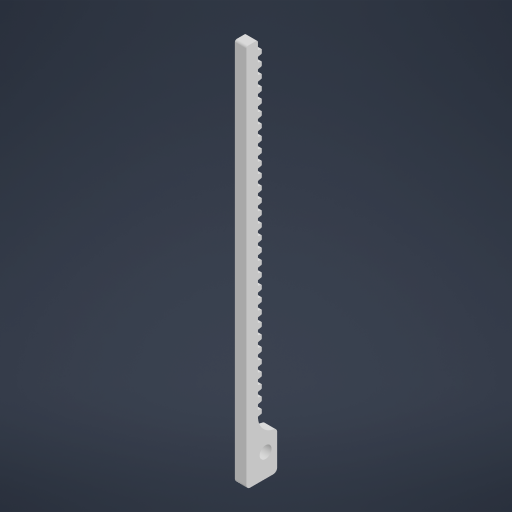
# Autodesk Inventor part: CamPole
Saved by Autodesk Inventor 2023 (Build 270158000, 158)
## iProperties
Created: 2023-03-14
Part Number: CamPole
Material: Generic
Document SubType Name: Modeling
Designer: Matt
Density: 1 g/cm^3
Appearance: Default
Author: Matt
Autodesk Inventor part; units mm, degrees
ref_plane "YZ Plane" through (0, 0, 0) normal (1, 0, 0) x (0, 1, 0)
ref_plane "XZ Plane" through (0, 0, 0) normal (0, 1, 0) x (-1, 0, 0)
ref_plane "XY Plane" through (0, 0, 0) normal (0, 0, 1) x (1, 0, 0)
sketch "Sketch1" plane through (0, 0, 0) normal (1, 0, 0) x (0, 1, 0)
  line L0 (0, 0) -> (10, 0)
  line L1 (10, 0) -> (10, -8)
  line L2 (10, -8) -> (0, -8)
  line L3 (0, -8) -> (0, 0)
  line L4 (10, 0) -> (100, 0)
  line L5 (100, 0) -> (100, -3)
  line L6 (100, -3) -> (10, -3)
  line L7 (10, -3) -> (10, 0)
  circle A0 centre (6, -5) radius 1.55
  dimension "d0" = 10
  dimension "d1" = 8
  dimension "d2" = 90
  dimension "d3" = 3
  dimension "d6" = 3.1
  dimension "d7" = 5
  dimension "d8" = 4
  constraints: 16 end point, 4 parallel, 2 horizontal, 2 perpendicular, 1 centre point
  measures "d0" distance of L1.end L2.end
  measures "d1" distance of L0.end L1.end
  measures "d2" distance of L0.end L4.end
  measures "d3" distance of L4.end L5.end
  measures "d6" diameter of A0
  measures "d7" distance from line of L0 A0.centre
  measures "d8" distance from line of L1 A0.centre
extrude "Extrusion1" add sketch "Sketch1" along normal blind 3
fillet "Fillet1" radius 5 1 edges at (1.5, 10, -3)
fillet "Fillet1" radius 1 3 edges at (1.5, 10, -8) (1.5, 0, 0) (1.5, 0, -8)
fillet "Fillet1" radius 0.5 2 edges at (1.5, 100, -3) (1.5, 100, 0)
sketch "Sketch3" plane through (3, 0, 0) normal (1, 0, 0) x (0, 0, -1)
  arc A0 (3, 15) -> (7.1667, 10.0699) centre (8, 15) ccw projected
  line L0 (3, 15) -> (4, 15)
  line L1 (4, 15) -> (4, 15.75)
  line L2 (4, 15.75) -> (3, 15.75)
  line L3 (3, 15) -> (3, 99.5) projected
  line L4 (3, 15) -> (3, 15.75)
  line L5 (4, 15) -> (4, 15.2)
  line L6 (4, 15.2) -> (3, 15)
  line L7 (3, 15) -> (3.1, 15)
  line L8 (3.1, 15) -> (3.1, 14.9)
  line L9 (3.1, 14.9) -> (3, 14.9)
  line L10 (3, 14.9) -> (3, 15)
  arc A1 (3.0995, 15.0199) -> (3, 14.9) centre (3.1238, 14.8985) ccw
  arc A2 (3.899, 15.1798) -> (4, 15.3306) centre (3.837, 15.3306) ccw
  line L11 (4, 15.3306) -> (4, 15.75)
  line L12 (3, 14.9) -> (3, 15.75)
  line L13 (3.899, 15.1798) -> (3.0995, 15.0199)
  line L14 (3, 16.5) -> (3, 15.75)
  line L15 (3, 16.6) -> (3, 16.5)
  arc A3 (3, 16.6) -> (3.0995, 16.4801) centre (3.1238, 16.6015) ccw
  arc A4 (4, 16.1694) -> (3.899, 16.3202) centre (3.837, 16.1694) ccw
  line L16 (4, 16.1694) -> (4, 15.75)
  line L17 (3.899, 16.3202) -> (3.0995, 16.4801)
  line L18 (4, 18.9694) -> (4, 18.55)
  arc A5 (3.899, 17.9798) -> (4, 18.1306) centre (3.837, 18.1306) ccw
  line L19 (3.899, 19.1202) -> (3.0995, 19.2801)
  arc A6 (4, 18.9694) -> (3.899, 19.1202) centre (3.837, 18.9694) ccw
  arc A7 (3, 19.4) -> (3.0995, 19.2801) centre (3.1238, 19.4015) ccw
  line L20 (3, 19.3) -> (3, 18.55)
  line L21 (3, 19.4) -> (3, 19.3)
  line L22 (3, 17.8) -> (3, 18.55)
  line L23 (3, 17.7) -> (3, 18.55)
  arc A8 (3.0995, 17.8199) -> (3, 17.7) centre (3.1238, 17.6985) ccw
  line L24 (4, 18.1306) -> (4, 18.55)
  line L25 (3.899, 17.9798) -> (3.0995, 17.8199)
  line L26 (4, 21.7694) -> (4, 21.35)
  arc A9 (3.899, 20.7798) -> (4, 20.9306) centre (3.837, 20.9306) ccw
  line L27 (3.899, 21.9202) -> (3.0995, 22.0801)
  arc A10 (4, 21.7694) -> (3.899, 21.9202) centre (3.837, 21.7694) ccw
  arc A11 (3, 22.2) -> (3.0995, 22.0801) centre (3.1238, 22.2015) ccw
  line L28 (3, 22.1) -> (3, 21.35)
  line L29 (3, 22.2) -> (3, 22.1)
  line L30 (3, 20.6) -> (3, 21.35)
  line L31 (3, 20.5) -> (3, 21.35)
  arc A12 (3.0995, 20.6199) -> (3, 20.5) centre (3.1238, 20.4985) ccw
  line L32 (4, 20.9306) -> (4, 21.35)
  line L33 (3.899, 20.7798) -> (3.0995, 20.6199)
  line L34 (4, 24.5694) -> (4, 24.15)
  arc A13 (3.899, 23.5798) -> (4, 23.7306) centre (3.837, 23.7306) ccw
  line L35 (3.899, 24.7202) -> (3.0995, 24.8801)
  arc A14 (4, 24.5694) -> (3.899, 24.7202) centre (3.837, 24.5694) ccw
  arc A15 (3, 25) -> (3.0995, 24.8801) centre (3.1238, 25.0015) ccw
  line L36 (3, 24.9) -> (3, 24.15)
  line L37 (3, 25) -> (3, 24.9)
  line L38 (3, 23.4) -> (3, 24.15)
  line L39 (3, 23.3) -> (3, 24.15)
  arc A16 (3.0995, 23.4199) -> (3, 23.3) centre (3.1238, 23.2985) ccw
  line L40 (4, 23.7306) -> (4, 24.15)
  line L41 (3.899, 23.5798) -> (3.0995, 23.4199)
  line L42 (4, 27.3694) -> (4, 26.95)
  arc A17 (3.899, 26.3798) -> (4, 26.5306) centre (3.837, 26.5306) ccw
  line L43 (3.899, 27.5202) -> (3.0995, 27.6801)
  arc A18 (4, 27.3694) -> (3.899, 27.5202) centre (3.837, 27.3694) ccw
  arc A19 (3, 27.8) -> (3.0995, 27.6801) centre (3.1238, 27.8015) ccw
  line L44 (3, 27.7) -> (3, 26.95)
  line L45 (3, 27.8) -> (3, 27.7)
  line L46 (3, 26.2) -> (3, 26.95)
  line L47 (3, 26.1) -> (3, 26.95)
  arc A20 (3.0995, 26.2199) -> (3, 26.1) centre (3.1238, 26.0985) ccw
  line L48 (4, 26.5306) -> (4, 26.95)
  line L49 (3.899, 26.3798) -> (3.0995, 26.2199)
  line L50 (4, 30.1694) -> (4, 29.75)
  arc A21 (3.899, 29.1798) -> (4, 29.3306) centre (3.837, 29.3306) ccw
  line L51 (3.899, 30.3202) -> (3.0995, 30.4801)
  arc A22 (4, 30.1694) -> (3.899, 30.3202) centre (3.837, 30.1694) ccw
  arc A23 (3, 30.6) -> (3.0995, 30.4801) centre (3.1238, 30.6015) ccw
  line L52 (3, 30.5) -> (3, 29.75)
  line L53 (3, 30.6) -> (3, 30.5)
  line L54 (3, 29) -> (3, 29.75)
  line L55 (3, 28.9) -> (3, 29.75)
  arc A24 (3.0995, 29.0199) -> (3, 28.9) centre (3.1238, 28.8985) ccw
  line L56 (4, 29.3306) -> (4, 29.75)
  line L57 (3.899, 29.1798) -> (3.0995, 29.0199)
  line L58 (4, 32.9694) -> (4, 32.55)
  arc A25 (3.899, 31.9798) -> (4, 32.1306) centre (3.837, 32.1306) ccw
  line L59 (3.899, 33.1202) -> (3.0995, 33.2801)
  arc A26 (4, 32.9694) -> (3.899, 33.1202) centre (3.837, 32.9694) ccw
  arc A27 (3, 33.4) -> (3.0995, 33.2801) centre (3.1238, 33.4015) ccw
  line L60 (3, 33.3) -> (3, 32.55)
  line L61 (3, 33.4) -> (3, 33.3)
  line L62 (3, 31.8) -> (3, 32.55)
  line L63 (3, 31.7) -> (3, 32.55)
  arc A28 (3.0995, 31.8199) -> (3, 31.7) centre (3.1238, 31.6985) ccw
  line L64 (4, 32.1306) -> (4, 32.55)
  line L65 (3.899, 31.9798) -> (3.0995, 31.8199)
  line L66 (4, 35.7694) -> (4, 35.35)
  arc A29 (3.899, 34.7798) -> (4, 34.9306) centre (3.837, 34.9306) ccw
  line L67 (3.899, 35.9202) -> (3.0995, 36.0801)
  arc A30 (4, 35.7694) -> (3.899, 35.9202) centre (3.837, 35.7694) ccw
  arc A31 (3, 36.2) -> (3.0995, 36.0801) centre (3.1238, 36.2015) ccw
  line L68 (3, 36.1) -> (3, 35.35)
  line L69 (3, 36.2) -> (3, 36.1)
  line L70 (3, 34.6) -> (3, 35.35)
  line L71 (3, 34.5) -> (3, 35.35)
  arc A32 (3.0995, 34.6199) -> (3, 34.5) centre (3.1238, 34.4985) ccw
  line L72 (4, 34.9306) -> (4, 35.35)
  line L73 (3.899, 34.7798) -> (3.0995, 34.6199)
  line L74 (4, 38.5694) -> (4, 38.15)
  arc A33 (3.899, 37.5798) -> (4, 37.7306) centre (3.837, 37.7306) ccw
  line L75 (3.899, 38.7202) -> (3.0995, 38.8801)
  arc A34 (4, 38.5694) -> (3.899, 38.7202) centre (3.837, 38.5694) ccw
  arc A35 (3, 39) -> (3.0995, 38.8801) centre (3.1238, 39.0015) ccw
  line L76 (3, 38.9) -> (3, 38.15)
  line L77 (3, 39) -> (3, 38.9)
  line L78 (3, 37.4) -> (3, 38.15)
  line L79 (3, 37.3) -> (3, 38.15)
  arc A36 (3.0995, 37.4199) -> (3, 37.3) centre (3.1238, 37.2985) ccw
  line L80 (4, 37.7306) -> (4, 38.15)
  line L81 (3.899, 37.5798) -> (3.0995, 37.4199)
  line L82 (4, 41.3694) -> (4, 40.95)
  arc A37 (3.899, 40.3798) -> (4, 40.5306) centre (3.837, 40.5306) ccw
  line L83 (3.899, 41.5202) -> (3.0995, 41.6801)
  arc A38 (4, 41.3694) -> (3.899, 41.5202) centre (3.837, 41.3694) ccw
  arc A39 (3, 41.8) -> (3.0995, 41.6801) centre (3.1238, 41.8015) ccw
  line L84 (3, 41.7) -> (3, 40.95)
  line L85 (3, 41.8) -> (3, 41.7)
  line L86 (3, 40.2) -> (3, 40.95)
  line L87 (3, 40.1) -> (3, 40.95)
  arc A40 (3.0995, 40.2199) -> (3, 40.1) centre (3.1238, 40.0985) ccw
  line L88 (4, 40.5306) -> (4, 40.95)
  line L89 (3.899, 40.3798) -> (3.0995, 40.2199)
  line L90 (4, 44.1694) -> (4, 43.75)
  arc A41 (3.899, 43.1798) -> (4, 43.3306) centre (3.837, 43.3306) ccw
  line L91 (3.899, 44.3202) -> (3.0995, 44.4801)
  arc A42 (4, 44.1694) -> (3.899, 44.3202) centre (3.837, 44.1694) ccw
  arc A43 (3, 44.6) -> (3.0995, 44.4801) centre (3.1238, 44.6015) ccw
  line L92 (3, 44.5) -> (3, 43.75)
  line L93 (3, 44.6) -> (3, 44.5)
  line L94 (3, 43) -> (3, 43.75)
  line L95 (3, 42.9) -> (3, 43.75)
  arc A44 (3.0995, 43.0199) -> (3, 42.9) centre (3.1238, 42.8985) ccw
  line L96 (4, 43.3306) -> (4, 43.75)
  line L97 (3.899, 43.1798) -> (3.0995, 43.0199)
  line L98 (4, 46.9694) -> (4, 46.55)
  arc A45 (3.899, 45.9798) -> (4, 46.1306) centre (3.837, 46.1306) ccw
  line L99 (3.899, 47.1202) -> (3.0995, 47.2801)
  arc A46 (4, 46.9694) -> (3.899, 47.1202) centre (3.837, 46.9694) ccw
  arc A47 (3, 47.4) -> (3.0995, 47.2801) centre (3.1238, 47.4015) ccw
  line L100 (3, 47.3) -> (3, 46.55)
  line L101 (3, 47.4) -> (3, 47.3)
  line L102 (3, 45.8) -> (3, 46.55)
  line L103 (3, 45.7) -> (3, 46.55)
  arc A48 (3.0995, 45.8199) -> (3, 45.7) centre (3.1238, 45.6985) ccw
  line L104 (4, 46.1306) -> (4, 46.55)
  line L105 (3.899, 45.9798) -> (3.0995, 45.8199)
  line L106 (4, 49.7694) -> (4, 49.35)
  arc A49 (3.899, 48.7798) -> (4, 48.9306) centre (3.837, 48.9306) ccw
  line L107 (3.899, 49.9202) -> (3.0995, 50.0801)
  arc A50 (4, 49.7694) -> (3.899, 49.9202) centre (3.837, 49.7694) ccw
  arc A51 (3, 50.2) -> (3.0995, 50.0801) centre (3.1238, 50.2015) ccw
  line L108 (3, 50.1) -> (3, 49.35)
  line L109 (3, 50.2) -> (3, 50.1)
  line L110 (3, 48.6) -> (3, 49.35)
  line L111 (3, 48.5) -> (3, 49.35)
  arc A52 (3.0995, 48.6199) -> (3, 48.5) centre (3.1238, 48.4985) ccw
  line L112 (4, 48.9306) -> (4, 49.35)
  line L113 (3.899, 48.7798) -> (3.0995, 48.6199)
  line L114 (4, 52.5694) -> (4, 52.15)
  arc A53 (3.899, 51.5798) -> (4, 51.7306) centre (3.837, 51.7306) ccw
  line L115 (3.899, 52.7202) -> (3.0995, 52.8801)
  arc A54 (4, 52.5694) -> (3.899, 52.7202) centre (3.837, 52.5694) ccw
  arc A55 (3, 53) -> (3.0995, 52.8801) centre (3.1238, 53.0015) ccw
  line L116 (3, 52.9) -> (3, 52.15)
  line L117 (3, 53) -> (3, 52.9)
  line L118 (3, 51.4) -> (3, 52.15)
  line L119 (3, 51.3) -> (3, 52.15)
  arc A56 (3.0995, 51.4199) -> (3, 51.3) centre (3.1238, 51.2985) ccw
  line L120 (4, 51.7306) -> (4, 52.15)
  line L121 (3.899, 51.5798) -> (3.0995, 51.4199)
  line L122 (4, 55.3694) -> (4, 54.95)
  arc A57 (3.899, 54.3798) -> (4, 54.5306) centre (3.837, 54.5306) ccw
  line L123 (3.899, 55.5202) -> (3.0995, 55.6801)
  arc A58 (4, 55.3694) -> (3.899, 55.5202) centre (3.837, 55.3694) ccw
  arc A59 (3, 55.8) -> (3.0995, 55.6801) centre (3.1238, 55.8015) ccw
  line L124 (3, 55.7) -> (3, 54.95)
  line L125 (3, 55.8) -> (3, 55.7)
  line L126 (3, 54.2) -> (3, 54.95)
  line L127 (3, 54.1) -> (3, 54.95)
  arc A60 (3.0995, 54.2199) -> (3, 54.1) centre (3.1238, 54.0985) ccw
  line L128 (4, 54.5306) -> (4, 54.95)
  line L129 (3.899, 54.3798) -> (3.0995, 54.2199)
  line L130 (4, 58.1694) -> (4, 57.75)
  arc A61 (3.899, 57.1798) -> (4, 57.3306) centre (3.837, 57.3306) ccw
  line L131 (3.899, 58.3202) -> (3.0995, 58.4801)
  arc A62 (4, 58.1694) -> (3.899, 58.3202) centre (3.837, 58.1694) ccw
  arc A63 (3, 58.6) -> (3.0995, 58.4801) centre (3.1238, 58.6015) ccw
  line L132 (3, 58.5) -> (3, 57.75)
  line L133 (3, 58.6) -> (3, 58.5)
  line L134 (3, 57) -> (3, 57.75)
  line L135 (3, 56.9) -> (3, 57.75)
  arc A64 (3.0995, 57.0199) -> (3, 56.9) centre (3.1238, 56.8985) ccw
  line L136 (4, 57.3306) -> (4, 57.75)
  line L137 (3.899, 57.1798) -> (3.0995, 57.0199)
  line L138 (4, 60.9694) -> (4, 60.55)
  arc A65 (3.899, 59.9798) -> (4, 60.1306) centre (3.837, 60.1306) ccw
  line L139 (3.899, 61.1202) -> (3.0995, 61.2801)
  arc A66 (4, 60.9694) -> (3.899, 61.1202) centre (3.837, 60.9694) ccw
  arc A67 (3, 61.4) -> (3.0995, 61.2801) centre (3.1238, 61.4015) ccw
  line L140 (3, 61.3) -> (3, 60.55)
  line L141 (3, 61.4) -> (3, 61.3)
  line L142 (3, 59.8) -> (3, 60.55)
  line L143 (3, 59.7) -> (3, 60.55)
  arc A68 (3.0995, 59.8199) -> (3, 59.7) centre (3.1238, 59.6985) ccw
  line L144 (4, 60.1306) -> (4, 60.55)
  line L145 (3.899, 59.9798) -> (3.0995, 59.8199)
  line L146 (4, 63.7694) -> (4, 63.35)
  arc A69 (3.899, 62.7798) -> (4, 62.9306) centre (3.837, 62.9306) ccw
  line L147 (3.899, 63.9202) -> (3.0995, 64.0801)
  arc A70 (4, 63.7694) -> (3.899, 63.9202) centre (3.837, 63.7694) ccw
  arc A71 (3, 64.2) -> (3.0995, 64.0801) centre (3.1238, 64.2015) ccw
  line L148 (3, 64.1) -> (3, 63.35)
  line L149 (3, 64.2) -> (3, 64.1)
  line L150 (3, 62.6) -> (3, 63.35)
  line L151 (3, 62.5) -> (3, 63.35)
  arc A72 (3.0995, 62.6199) -> (3, 62.5) centre (3.1238, 62.4985) ccw
  line L152 (4, 62.9306) -> (4, 63.35)
  line L153 (3.899, 62.7798) -> (3.0995, 62.6199)
  line L154 (4, 66.5694) -> (4, 66.15)
  arc A73 (3.899, 65.5798) -> (4, 65.7306) centre (3.837, 65.7306) ccw
  line L155 (3.899, 66.7202) -> (3.0995, 66.8801)
  arc A74 (4, 66.5694) -> (3.899, 66.7202) centre (3.837, 66.5694) ccw
  arc A75 (3, 67) -> (3.0995, 66.8801) centre (3.1238, 67.0015) ccw
  line L156 (3, 66.9) -> (3, 66.15)
  line L157 (3, 67) -> (3, 66.9)
  line L158 (3, 65.4) -> (3, 66.15)
  line L159 (3, 65.3) -> (3, 66.15)
  arc A76 (3.0995, 65.4199) -> (3, 65.3) centre (3.1238, 65.2985) ccw
  line L160 (4, 65.7306) -> (4, 66.15)
  line L161 (3.899, 65.5798) -> (3.0995, 65.4199)
  line L162 (4, 69.3694) -> (4, 68.95)
  arc A77 (3.899, 68.3798) -> (4, 68.5306) centre (3.837, 68.5306) ccw
  line L163 (3.899, 69.5202) -> (3.0995, 69.6801)
  arc A78 (4, 69.3694) -> (3.899, 69.5202) centre (3.837, 69.3694) ccw
  arc A79 (3, 69.8) -> (3.0995, 69.6801) centre (3.1238, 69.8015) ccw
  line L164 (3, 69.7) -> (3, 68.95)
  line L165 (3, 69.8) -> (3, 69.7)
  line L166 (3, 68.2) -> (3, 68.95)
  line L167 (3, 68.1) -> (3, 68.95)
  arc A80 (3.0995, 68.2199) -> (3, 68.1) centre (3.1238, 68.0985) ccw
  line L168 (4, 68.5306) -> (4, 68.95)
  line L169 (3.899, 68.3798) -> (3.0995, 68.2199)
  line L170 (4, 72.1694) -> (4, 71.75)
  arc A81 (3.899, 71.1798) -> (4, 71.3306) centre (3.837, 71.3306) ccw
  line L171 (3.899, 72.3202) -> (3.0995, 72.4801)
  arc A82 (4, 72.1694) -> (3.899, 72.3202) centre (3.837, 72.1694) ccw
  arc A83 (3, 72.6) -> (3.0995, 72.4801) centre (3.1238, 72.6015) ccw
  line L172 (3, 72.5) -> (3, 71.75)
  line L173 (3, 72.6) -> (3, 72.5)
  line L174 (3, 71) -> (3, 71.75)
  line L175 (3, 70.9) -> (3, 71.75)
  arc A84 (3.0995, 71.0199) -> (3, 70.9) centre (3.1238, 70.8985) ccw
  line L176 (4, 71.3306) -> (4, 71.75)
  line L177 (3.899, 71.1798) -> (3.0995, 71.0199)
  line L178 (4, 74.9694) -> (4, 74.55)
  arc A85 (3.899, 73.9798) -> (4, 74.1306) centre (3.837, 74.1306) ccw
  line L179 (3.899, 75.1202) -> (3.0995, 75.2801)
  arc A86 (4, 74.9694) -> (3.899, 75.1202) centre (3.837, 74.9694) ccw
  arc A87 (3, 75.4) -> (3.0995, 75.2801) centre (3.1238, 75.4015) ccw
  line L180 (3, 75.3) -> (3, 74.55)
  line L181 (3, 75.4) -> (3, 75.3)
  line L182 (3, 73.8) -> (3, 74.55)
  line L183 (3, 73.7) -> (3, 74.55)
  arc A88 (3.0995, 73.8199) -> (3, 73.7) centre (3.1238, 73.6985) ccw
  line L184 (4, 74.1306) -> (4, 74.55)
  line L185 (3.899, 73.9798) -> (3.0995, 73.8199)
  line L186 (4, 77.7694) -> (4, 77.35)
  arc A89 (3.899, 76.7798) -> (4, 76.9306) centre (3.837, 76.9306) ccw
  line L187 (3.899, 77.9202) -> (3.0995, 78.0801)
  arc A90 (4, 77.7694) -> (3.899, 77.9202) centre (3.837, 77.7694) ccw
  arc A91 (3, 78.2) -> (3.0995, 78.0801) centre (3.1238, 78.2015) ccw
  line L188 (3, 78.1) -> (3, 77.35)
  line L189 (3, 78.2) -> (3, 78.1)
  line L190 (3, 76.6) -> (3, 77.35)
  line L191 (3, 76.5) -> (3, 77.35)
  arc A92 (3.0995, 76.6199) -> (3, 76.5) centre (3.1238, 76.4985) ccw
  line L192 (4, 76.9306) -> (4, 77.35)
  line L193 (3.899, 76.7798) -> (3.0995, 76.6199)
  line L194 (4, 80.5694) -> (4, 80.15)
  arc A93 (3.899, 79.5798) -> (4, 79.7306) centre (3.837, 79.7306) ccw
  line L195 (3.899, 80.7202) -> (3.0995, 80.8801)
  arc A94 (4, 80.5694) -> (3.899, 80.7202) centre (3.837, 80.5694) ccw
  arc A95 (3, 81) -> (3.0995, 80.8801) centre (3.1238, 81.0015) ccw
  line L196 (3, 80.9) -> (3, 80.15)
  line L197 (3, 81) -> (3, 80.9)
  line L198 (3, 79.4) -> (3, 80.15)
  line L199 (3, 79.3) -> (3, 80.15)
  arc A96 (3.0995, 79.4199) -> (3, 79.3) centre (3.1238, 79.2985) ccw
  line L200 (4, 79.7306) -> (4, 80.15)
  line L201 (3.899, 79.5798) -> (3.0995, 79.4199)
  line L202 (4, 83.3694) -> (4, 82.95)
  arc A97 (3.899, 82.3798) -> (4, 82.5306) centre (3.837, 82.5306) ccw
  line L203 (3.899, 83.5202) -> (3.0995, 83.6801)
  arc A98 (4, 83.3694) -> (3.899, 83.5202) centre (3.837, 83.3694) ccw
  arc A99 (3, 83.8) -> (3.0995, 83.6801) centre (3.1238, 83.8015) ccw
  line L204 (3, 83.7) -> (3, 82.95)
  line L205 (3, 83.8) -> (3, 83.7)
  line L206 (3, 82.2) -> (3, 82.95)
  line L207 (3, 82.1) -> (3, 82.95)
  arc A100 (3.0995, 82.2199) -> (3, 82.1) centre (3.1238, 82.0985) ccw
  line L208 (4, 82.5306) -> (4, 82.95)
  line L209 (3.899, 82.3798) -> (3.0995, 82.2199)
  line L210 (4, 86.1694) -> (4, 85.75)
  arc A101 (3.899, 85.1798) -> (4, 85.3306) centre (3.837, 85.3306) ccw
  line L211 (3.899, 86.3202) -> (3.0995, 86.4801)
  arc A102 (4, 86.1694) -> (3.899, 86.3202) centre (3.837, 86.1694) ccw
  arc A103 (3, 86.6) -> (3.0995, 86.4801) centre (3.1238, 86.6015) ccw
  line L212 (3, 86.5) -> (3, 85.75)
  line L213 (3, 86.6) -> (3, 86.5)
  line L214 (3, 85) -> (3, 85.75)
  line L215 (3, 84.9) -> (3, 85.75)
  arc A104 (3.0995, 85.0199) -> (3, 84.9) centre (3.1238, 84.8985) ccw
  line L216 (4, 85.3306) -> (4, 85.75)
  line L217 (3.899, 85.1798) -> (3.0995, 85.0199)
  line L218 (4, 88.9694) -> (4, 88.55)
  arc A105 (3.899, 87.9798) -> (4, 88.1306) centre (3.837, 88.1306) ccw
  line L219 (3.899, 89.1202) -> (3.0995, 89.2801)
  arc A106 (4, 88.9694) -> (3.899, 89.1202) centre (3.837, 88.9694) ccw
  arc A107 (3, 89.4) -> (3.0995, 89.2801) centre (3.1238, 89.4015) ccw
  line L220 (3, 89.3) -> (3, 88.55)
  line L221 (3, 89.4) -> (3, 89.3)
  line L222 (3, 87.8) -> (3, 88.55)
  line L223 (3, 87.7) -> (3, 88.55)
  arc A108 (3.0995, 87.8199) -> (3, 87.7) centre (3.1238, 87.6985) ccw
  line L224 (4, 88.1306) -> (4, 88.55)
  line L225 (3.899, 87.9798) -> (3.0995, 87.8199)
  line L226 (4, 91.7694) -> (4, 91.35)
  arc A109 (3.899, 90.7798) -> (4, 90.9306) centre (3.837, 90.9306) ccw
  line L227 (3.899, 91.9202) -> (3.0995, 92.0801)
  arc A110 (4, 91.7694) -> (3.899, 91.9202) centre (3.837, 91.7694) ccw
  arc A111 (3, 92.2) -> (3.0995, 92.0801) centre (3.1238, 92.2015) ccw
  line L228 (3, 92.1) -> (3, 91.35)
  line L229 (3, 92.2) -> (3, 92.1)
  line L230 (3, 90.6) -> (3, 91.35)
  line L231 (3, 90.5) -> (3, 91.35)
  arc A112 (3.0995, 90.6199) -> (3, 90.5) centre (3.1238, 90.4985) ccw
  line L232 (4, 90.9306) -> (4, 91.35)
  line L233 (3.899, 90.7798) -> (3.0995, 90.6199)
  line L234 (4, 94.5694) -> (4, 94.15)
  arc A113 (3.899, 93.5798) -> (4, 93.7306) centre (3.837, 93.7306) ccw
  line L235 (3.899, 94.7202) -> (3.0995, 94.8801)
  arc A114 (4, 94.5694) -> (3.899, 94.7202) centre (3.837, 94.5694) ccw
  arc A115 (3, 95) -> (3.0995, 94.8801) centre (3.1238, 95.0015) ccw
  line L236 (3, 94.9) -> (3, 94.15)
  line L237 (3, 95) -> (3, 94.9)
  line L238 (3, 93.4) -> (3, 94.15)
  line L239 (3, 93.3) -> (3, 94.15)
  arc A116 (3.0995, 93.4199) -> (3, 93.3) centre (3.1238, 93.2985) ccw
  line L240 (4, 93.7306) -> (4, 94.15)
  line L241 (3.899, 93.5798) -> (3.0995, 93.4199)
  line L242 (4, 97.3694) -> (4, 96.95)
  arc A117 (3.899, 96.3798) -> (4, 96.5306) centre (3.837, 96.5306) ccw
  line L243 (3.899, 97.5202) -> (3.0995, 97.6801)
  arc A118 (4, 97.3694) -> (3.899, 97.5202) centre (3.837, 97.3694) ccw
  arc A119 (3, 97.8) -> (3.0995, 97.6801) centre (3.1238, 97.8015) ccw
  line L244 (3, 97.7) -> (3, 96.95)
  line L245 (3, 97.8) -> (3, 97.7)
  line L246 (3, 96.2) -> (3, 96.95)
  line L247 (3, 96.1) -> (3, 96.95)
  arc A120 (3.0995, 96.2199) -> (3, 96.1) centre (3.1238, 96.0985) ccw
  line L248 (4, 96.5306) -> (4, 96.95)
  line L249 (3.899, 96.3798) -> (3.0995, 96.2199)
  point P0 (0, 0)
  point P1 (3, 97.8)
  point P2 (3, 96.1)
  point P3 (3, 55.8)
  point P4 (3, 54.1)
  point P5 (3, 58.6)
  point P6 (3, 56.9)
  point P7 (3, 53)
  point P8 (3, 51.3)
  point P9 (3, 61.4)
  point P10 (3, 59.7)
  point P11 (3, 50.2)
  point P12 (3, 48.5)
  point P13 (3, 64.2)
  point P14 (3, 62.5)
  point P15 (3, 67)
  point P16 (3, 65.3)
  point P17 (3, 69.8)
  point P18 (3, 68.1)
  point P19 (3, 72.6)
  point P20 (3, 70.9)
  point P21 (3, 75.4)
  point P22 (3, 73.7)
  point P23 (3, 78.2)
  point P24 (3, 76.5)
  point P25 (3, 81)
  point P26 (3, 79.3)
  point P27 (3, 83.8)
  point P28 (3, 82.1)
  point P29 (3, 86.6)
  point P30 (3, 84.9)
  point P31 (3, 89.4)
  point P32 (3, 87.7)
  point P33 (3, 92.2)
  point P34 (3, 90.5)
  point P35 (3, 95)
  point P36 (3, 93.3)
  point P37 (3, 47.4)
  point P38 (3, 45.7)
  point P39 (3, 22.2)
  point P40 (3, 20.5)
  point P41 (3, 44.6)
  point P42 (3, 42.9)
  point P43 (3, 19.4)
  point P44 (3, 17.7)
  point P45 (3, 41.8)
  point P46 (3, 40.1)
  point P47 (3, 39)
  point P48 (3, 37.3)
  point P49 (3, 36.2)
  point P50 (3, 34.5)
  point P51 (3, 33.4)
  point P52 (3, 31.7)
  point P53 (3, 30.6)
  point P54 (3, 28.9)
  point P55 (3, 27.8)
  point P56 (3, 26.1)
  point P57 (3, 25)
  point P58 (3, 23.3)
  point P59 (3, 16.6)
  point P60 (3.001, 14.9)
  point P61 (3.0008, 14.9123)
  dimension "d12" = 1
  dimension "d13" = 0.75
  dimension "d14" = 0.2
  dimension "d15" = 0.1
  dimension "d16" = 0.1
  dimension "d19" = 2.8
  constraints: 498 end point, 464 vertical alignment, 240 point on circle, 176 collinear, 120 centre point, 116 equal radius, 60 parallel, 7 symmetric about line, 4 perpendicular, 4 point on line, 2 horizontal, 2 tangent, 1 vertical, 4 other
  measures "d12" distance of L0.start L0.end
  measures "d13" distance of L0.end L1.end
  measures "d14" distance of L0.end L5.end
  measures "d15" distance of L8.end L9.end
  measures "d16" distance of L7.end L8.end
  measures "d19" distance of L16.start L18.start
extrude "Extrusion2" add sketch "Sketch3" against normal up to surface (3 mm away) contours L0 A1 A0 | L6 A1 L0 | L3 L2 L1 A2 L6 | L3 A3 L17 A4 L16 L2 | L3 A7 L19 A6 L18 L24 A5 L25 A8 | L3 A11 L27 A10 L26 L32 A9 L33 A12 | L3 A15 L35 A14 L34 L40 A13 L41 A16 | L3 A19 L43 A18 L42 L48 A17 L49 A20 | L3 A23 L51 A22 L50 L56 A21 L57 A24 | L3 A27 L59 A26 L58 L64 A25 L65 A28 | L3 A31 L67 A30 L66 L72 A29 L73 A32 | L3 A35 L75 A34 L74 L80 A33 L81 A36 | L3 A39 L83 A38 L82 L88 A37 L89 A40 | L3 A43 L91 A42 L90 L96 A41 L97 A44 | L3 A47 L99 A46 L98 L104 A45 L105 A48 | L3 A51 L107 A50 L106 L112 A49 L113 A52 | L3 A55 L115 A54 L114 L120 A53 L121 A56 | L3 A59 L123 A58 L122 L128 A57 L129 A60 | L3 A63 L131 A62 L130 L136 A61 L137 A64 | L3 A67 L139 A66 L138 L144 A65 L145 A68 | L3 A71 L147 A70 L146 L152 A69 L153 A72 | L3 A75 L155 A74 L154 L160 A73 L161 A76 | L3 A79 L163 A78 L162 L168 A77 L169 A80 | L3 A83 L171 A82 L170 L176 A81 L177 A84 | L3 A87 L179 A86 L178 L184 A85 L185 A88 | L3 A91 L187 A90 L186 L192 A89 L193 A92 | L3 A95 L195 A94 L194 L200 A93 L201 A96 | L3 A99 L203 A98 L202 L208 A97 L209 A100 | L3 A103 L211 A102 L210 L216 A101 L217 A104 | L3 A107 L219 A106 L218 L224 A105 L225 A108 | L3 A111 L227 A110 L226 L232 A109 L233 A112 | L3 A115 L235 A114 L234 L240 A113 L241 A116 | L3 A119 L243 A118 L242 L248 A117 L249 A120
equation "\"Acrylic\" = 3"
body "Solid1"
